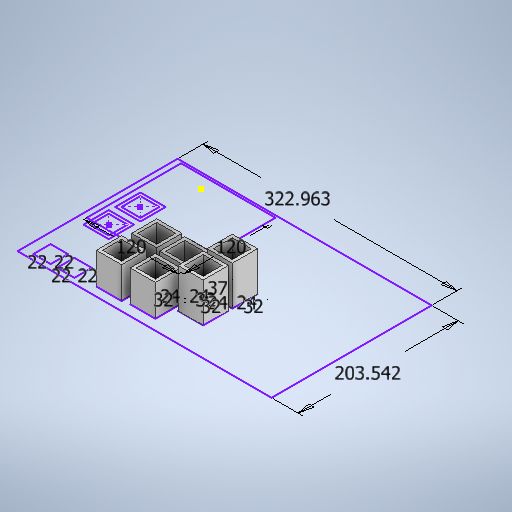
# Autodesk Inventor part: axie3
Saved by Autodesk Inventor 2025.1 (Build 291241000, 241)
## iProperties
Created: 2024-10-25
Part Number: axie3
Material: 一般
Document SubType Name: Modeling
Designer: youtian
Density: 1 g/cm^3
Appearance: 預設
Author: youtian
Autodesk Inventor part; units mm, degrees
ref_plane "YZ Plane" through (0, 0, 0) normal (1, 0, 0) x (0, 1, 0)
ref_plane "XZ Plane" through (0, 0, 0) normal (0, 1, 0) x (-1, 0, 0)
ref_plane "XY Plane" through (0, 0, 0) normal (0, 0, 1) x (1, 0, 0)
sketch "草圖1" plane through (0, 0, 0) normal (0, 1, 0) x (-1, 0, 0)
  circle A0 centre (0, 0) radius 7
  circle A1 centre (0, 0) radius 11
  line L0 (0, 0) -> (-26.517, 0)
  line L1 (0, 0) -> (0, 28.4195)
  circle A2 centre (-26, 0) radius 7
  circle A3 centre (-26, 0) radius 11
  circle A4 centre (0, 26) radius 7
  circle A5 centre (0, 26) radius 11
  circle A6 centre (-26, 26) radius 7
  circle A7 centre (-26, 26) radius 11
  dimension "d0" = 14
  dimension "d1" = 22
  dimension "d6" = 26
  dimension "d9" = 26
  constraints: 8 centre point, 5 coincident, 4 end point, 2 horizontal, 2 vertical, 12 other
  measures "d0" diameter of A0
  measures "d1" diameter of A1
  measures "d6" distance of A0.centre A2.centre
  measures "d9" distance of A0.centre A4.centre
sketch "草圖6" plane through (0, 0, 0) normal (0, 1, 0) x (-1, 0, 0)
  point P0 (0, 0)
sketch "草圖9" plane through (0, 0, 0) normal (0, 1, 0) x (-1, 0, 0)
  line L0 (-119.4877, 79.3379) -> (-151.4877, 79.3379)
  line L1 (-151.4877, 79.3379) -> (-151.4877, 111.3379)
  line L2 (-151.4877, 111.3379) -> (-119.4877, 111.3379)
  line L3 (-119.4877, 111.3379) -> (-119.4877, 79.3379)
  line L4 (-123.4877, 83.3379) -> (-147.4877, 83.3379)
  line L5 (-147.4877, 83.3379) -> (-147.4877, 107.3379)
  line L6 (-147.4877, 107.3379) -> (-123.4877, 107.3379)
  line L7 (-123.4877, 107.3379) -> (-123.4877, 83.3379)
  line L8 (-123.4877, 83.3379) -> (-147.4877, 107.3379) construction
  line L9 (-147.4877, 83.3379) -> (-123.4877, 107.3379) construction
  line L10 (-119.4877, 116.3379) -> (-151.4877, 116.3379)
  line L11 (-151.4877, 116.3379) -> (-151.4877, 148.3379)
  line L12 (-151.4877, 148.3379) -> (-119.4877, 148.3379)
  line L13 (-119.4877, 148.3379) -> (-119.4877, 116.3379)
  line L14 (-123.4877, 120.3379) -> (-147.4877, 120.3379)
  line L15 (-147.4877, 120.3379) -> (-147.4877, 144.3379)
  line L16 (-147.4877, 144.3379) -> (-123.4877, 144.3379)
  line L17 (-123.4877, 144.3379) -> (-123.4877, 120.3379)
  line L18 (-123.4877, 120.3379) -> (-147.4877, 144.3379) construction
  line L19 (-147.4877, 120.3379) -> (-123.4877, 144.3379) construction
  line L20 (-82.0628, 102.3085) -> (-114.0628, 102.3085)
  line L21 (-114.0628, 102.3085) -> (-114.0628, 134.3085)
  line L22 (-114.0628, 134.3085) -> (-82.0628, 134.3085)
  line L23 (-82.0628, 134.3085) -> (-82.0628, 102.3085)
  line L24 (-86.0628, 106.3085) -> (-110.0628, 106.3085)
  line L25 (-110.0628, 106.3085) -> (-110.0628, 130.3085)
  line L26 (-110.0628, 130.3085) -> (-86.0628, 130.3085)
  line L27 (-86.0628, 130.3085) -> (-86.0628, 106.3085)
  line L28 (-86.0628, 102.6348) -> (-110.0628, 126.6348) construction
  line L29 (-110.0628, 102.6348) -> (-86.0628, 126.6348) construction
  line L30 (35.5473, 81.3984) -> (3.5473, 81.3984)
  line L31 (3.5473, 81.3984) -> (3.5473, 113.3984)
  line L32 (3.5473, 113.3984) -> (35.5473, 113.3984)
  line L33 (35.5473, 113.3984) -> (35.5473, 81.3984)
  line L34 (31.5472, 85.3984) -> (7.5472, 85.3984)
  line L35 (7.5472, 85.3984) -> (7.5472, 109.3984)
  line L36 (7.5472, 109.3984) -> (31.5472, 109.3984)
  line L37 (31.5472, 109.3984) -> (31.5472, 85.3984)
  line L38 (31.5472, 85.3984) -> (7.5472, 109.3984) construction
  line L39 (7.5472, 85.3984) -> (31.5472, 109.3984) construction
  line L40 (34.8593, 41.843) -> (2.8593, 41.843)
  line L41 (30.8593, 45.843) -> (6.8593, 45.843)
  line L42 (6.8593, 45.843) -> (6.8593, 69.843)
  line L43 (2.8593, 41.843) -> (2.8593, 73.843)
  line L44 (6.8593, 69.843) -> (30.8593, 69.843)
  line L45 (30.8593, 45.843) -> (6.8593, 69.843) construction
  line L46 (6.8593, 45.843) -> (30.8593, 69.843) construction
  line L47 (2.8593, 73.843) -> (34.8593, 73.843)
  line L48 (30.8593, 69.843) -> (30.8593, 45.843)
  line L49 (34.8593, 73.843) -> (34.8593, 41.843)
  line L50 (-44.571, 100.4659) -> (-76.571, 100.4659)
  line L51 (-48.5711, 104.466) -> (-72.5711, 104.466)
  line L52 (-72.5711, 104.466) -> (-72.5711, 128.466)
  line L53 (-76.571, 100.4659) -> (-76.571, 132.4659)
  line L54 (-72.5711, 128.466) -> (-48.5711, 128.466)
  line L55 (-48.5711, 104.466) -> (-72.5711, 128.466) construction
  line L56 (-72.5711, 104.466) -> (-48.5711, 128.466) construction
  line L57 (-76.571, 132.4659) -> (-44.571, 132.4659)
  line L58 (-48.5711, 128.466) -> (-48.5711, 104.466)
  line L59 (-44.571, 132.4659) -> (-44.571, 100.4659)
  line L60 (-40.805, 141.4327) -> (-72.805, 141.4327)
  line L61 (-44.805, 145.4328) -> (-68.805, 145.4328)
  line L62 (-68.805, 145.4328) -> (-68.805, 169.4328)
  line L63 (-72.805, 141.4327) -> (-72.805, 173.4327)
  line L64 (-68.805, 169.4328) -> (-44.805, 169.4328)
  line L65 (-44.805, 145.4328) -> (-68.805, 169.4328) construction
  line L66 (-68.805, 145.4328) -> (-44.805, 169.4328) construction
  line L67 (-72.805, 173.4327) -> (-40.805, 173.4327)
  line L68 (-44.805, 169.4328) -> (-44.805, 145.4328)
  line L69 (-40.805, 173.4327) -> (-40.805, 141.4327)
  line L70 (-81.8163, 139.4435) -> (-113.8163, 139.4435)
  line L71 (-85.8164, 143.4436) -> (-109.8164, 143.4436)
  line L72 (-109.8164, 143.4436) -> (-109.8164, 167.4436)
  line L73 (-113.8163, 139.4435) -> (-113.8163, 171.4435)
  line L74 (-109.8164, 167.4436) -> (-85.8164, 167.4436)
  line L75 (-85.8164, 143.4436) -> (-109.8164, 167.4436) construction
  line L76 (-109.8164, 143.4436) -> (-85.8164, 167.4436) construction
  line L77 (-113.8163, 171.4435) -> (-81.8163, 171.4435)
  line L78 (-85.8164, 167.4436) -> (-85.8164, 143.4436)
  line L79 (-81.8163, 171.4435) -> (-81.8163, 139.4435)
  point P0 (0, 0)
  point P1 (-135.4877, 95.3379)
  point P2 (-135.4877, 132.3379)
  point P3 (-98.0628, 114.6348)
  point P4 (19.5472, 97.3984)
  point P5 (18.8593, 57.843)
  point P6 (-60.5711, 116.466)
  point P7 (-56.805, 157.4328)
  point P8 (-97.8164, 155.4436)
  dimension "d73" = 50.747
  dimension "d54" = 32
  dimension "d55" = 32
  dimension "d56" = 24
  dimension "d57" = 24
  dimension "d60" = 37
  dimension "d69" = 32
  dimension "d70" = 32
  dimension "d71" = 24
  dimension "d72" = 24
  constraints: 160 end point, 8 parallel, 4 horizontal, 4 midpoint, 4 perpendicular, 2 vertical, 1 collinear, 18 other
  measures "d54" distance of L1.end L2.end
  measures "d55" distance of L0.end L1.end
  measures "d56" distance of L5.end L6.end
  measures "d57" distance of L4.end L5.end
  measures "d60" distance of L0.start L10.start
  measures "d69" distance of L22.start L22.end
  measures "d70" distance of L20.end L22.start
  measures "d71" distance of L26.start L26.end
  measures "d72" distance of L24.end L26.start
extrude "擠出9" add sketch "草圖9" along normal blind 50 contours L0 L1 L2 L3 | L10 L11 L12 L13
extrude "擠出10" add sketch "草圖9" along normal blind 40 contours L20 L21 L22 L23 | L50 L53 L57 L59 | L60 L63 L67 L69 | L70 L73 L77 L79
sketch "草圖10" plane through (0, 0, 0) normal (0, 1, 0) x (-1, 0, 0)
  line L0 (48.2716, 184.5725) -> (-274.6912, 184.5725)
  line L1 (-274.6912, 184.5725) -> (-274.6912, -18.9692)
  line L2 (-274.6912, -18.9692) -> (48.2716, -18.9692)
  line L3 (48.2716, -18.9692) -> (48.2716, 184.5725)
  point P0 (0, 0)
  dimension "d99" = 322.9628
  dimension "d100" = 203.5417
  constraints: 8 end point, 2 parallel, 1 horizontal, 1 perpendicular
  measures "d99" distance of L1.end L2.end
  measures "d100" distance of L0.end L1.end
sketch "草圖11" plane through (0, 0, 0) normal (0, 1, 0) x (-1, 0, 0)
  line L0 (35.0654, 155.7952) -> (13.0654, 155.7952)
  line L1 (13.0654, 155.7952) -> (13.0654, 177.7952)
  line L2 (13.0654, 177.7952) -> (35.0654, 177.7952)
  line L3 (35.0654, 177.7952) -> (35.0654, 155.7952)
  line L4 (4.7905, 155.7952) -> (-17.2095, 155.7952)
  line L5 (-17.2095, 155.7952) -> (-17.2095, 177.7952)
  line L6 (-17.2095, 177.7952) -> (4.7905, 177.7952)
  line L7 (4.7905, 177.7952) -> (4.7905, 155.7952)
  point P0 (0, 0)
  dimension "d101" = 22
  dimension "d102" = 22
  dimension "d103" = 22
  dimension "d104" = 22
  constraints: 16 end point, 4 parallel, 2 horizontal, 2 perpendicular
  measures "d101" distance of L1.end L2.end
  measures "d102" distance of L0.end L1.end
  measures "d103" distance of L5.end L6.end
  measures "d104" distance of L4.end L5.end
sketch "草圖12" plane through (0, 0, 0) normal (0, 1, 0) x (-1, 0, 0)
  line L0 (-109.331, 73.1874) -> (-109.331, 93.1874)
  line L1 (-109.331, 93.1874) -> (-89.331, 93.1874)
  line L2 (-89.331, 93.1874) -> (-89.331, 73.1874)
  line L3 (-89.331, 73.1874) -> (-109.331, 73.1874)
  line L4 (-80.953, 73.904) -> (-80.953, 93.904)
  line L5 (-80.953, 93.904) -> (-60.953, 93.904)
  line L6 (-60.953, 93.904) -> (-60.953, 73.904)
  line L7 (-60.953, 73.904) -> (-80.953, 73.904)
  line L8 (-38.2379, 177.9784) -> (-158.2379, 177.9784)
  line L9 (-158.2379, 177.9784) -> (-158.2379, 57.9784)
  line L10 (-158.2379, 57.9784) -> (-38.2379, 57.9784)
  line L11 (-38.2379, 57.9784) -> (-38.2379, 177.9784)
  point P0 (0, 0)
  dimension "d105" = 20
  dimension "d106" = 20
  dimension "d107" = 20
  dimension "d108" = 20
  dimension "d137" = 120
  dimension "d138" = 120
  constraints: 24 end point, 6 parallel, 3 perpendicular, 1 horizontal
  measures "d105" distance of L1.end L2.end
  measures "d106" distance of L0.end L1.end
  measures "d107" distance of L5.end L6.end
  measures "d108" distance of L4.end L5.end
  measures "d137" distance of L10.end L9.end
  measures "d138" distance of L9.end L8.end
extrude "擠出12" add sketch "草圖12" along normal blind 12 contours L0 L1 L2 L3 | L4 L5 L6 L7
sketch "草圖13" plane through (0, 12, 0) normal (0, 1, 0) x (1, 0, 0)
  line L0 (60.953, -73.904) -> (60.953, -93.904) projected
  line L1 (80.953, -93.904) -> (80.953, -73.904) projected
  line L2 (60.953, -93.904) -> (80.953, -73.904)
  line L3 (89.331, -93.1874) -> (109.331, -93.1874) projected
  line L4 (109.331, -93.1874) -> (109.331, -73.1874) projected
  line L5 (89.331, -93.1874) -> (109.331, -73.1874)
  line L6 (-13.0654, -155.7952) -> (-35.0654, -155.7952) projected
  line L7 (-35.0654, -177.7952) -> (-13.0654, -177.7952) projected
  line L8 (-35.0654, -155.7952) -> (-13.0654, -177.7952)
  line L9 (-4.7905, -177.7952) -> (17.2095, -177.7952) projected
  line L10 (-4.7905, -155.7952) -> (17.2095, -177.7952)
  line L11 (-31.0654, -159.7952) -> (-17.0654, -159.7952)
  line L12 (-17.0654, -159.7952) -> (-17.0654, -173.7952)
  line L13 (-17.0654, -173.7952) -> (-31.0654, -173.7952)
  line L14 (-31.0654, -173.7952) -> (-31.0654, -159.7952)
  line L15 (-31.0654, -159.7952) -> (-17.0654, -173.7952) construction
  line L16 (-17.0654, -159.7952) -> (-31.0654, -173.7952) construction
  line L17 (-0.7905, -173.7952) -> (13.2095, -173.7952)
  line L18 (13.2095, -173.7952) -> (13.2095, -159.7952)
  line L19 (13.2095, -159.7952) -> (-0.7905, -159.7952)
  line L20 (-0.7905, -159.7952) -> (-0.7905, -173.7952)
  line L21 (-0.7905, -173.7952) -> (13.2095, -159.7952) construction
  line L22 (13.2095, -173.7952) -> (-0.7905, -159.7952) construction
  line L23 (65.853, -78.804) -> (76.053, -78.804)
  line L24 (76.053, -78.804) -> (76.053, -89.004)
  line L25 (76.053, -89.004) -> (65.853, -89.004)
  line L26 (65.853, -89.004) -> (65.853, -78.804)
  line L27 (65.853, -78.804) -> (76.053, -89.004) construction
  line L28 (76.053, -78.804) -> (65.853, -89.004) construction
  line L29 (94.231, -88.2874) -> (104.431, -88.2874)
  line L30 (104.431, -88.2874) -> (104.431, -78.0874)
  line L31 (104.431, -78.0874) -> (94.231, -78.0874)
  line L32 (94.231, -78.0874) -> (94.231, -88.2874)
  line L33 (94.231, -88.2874) -> (104.431, -78.0874) construction
  line L34 (104.431, -88.2874) -> (94.231, -78.0874) construction
  point P0 (0, 0)
  point P1 (-24.0654, -166.7952)
  point P2 (6.2095, -166.7952)
  point P3 (70.953, -83.904)
  point P4 (99.331, -83.1874)
  dimension "d113" = 14
  dimension "d114" = 14
  dimension "d115" = 14
  dimension "d116" = 14
  dimension "d117" = 10.2
  dimension "d118" = 10.2
  dimension "d119" = 10.2
  dimension "d120" = 10.2
  constraints: 56 end point, 12 midpoint, 8 parallel, 4 horizontal, 4 perpendicular
  measures "d113" distance of L12.end L13.end
  measures "d114" distance of L11.end L12.end
  measures "d115" distance of L19.end L18.end
  measures "d116" distance of L18.end L17.end
  measures "d117" distance of L24.end L25.end
  measures "d118" distance of L23.end L24.end
  measures "d119" distance of L31.end L30.end
  measures "d120" distance of L30.end L29.end
extrude "擠出13" cut sketch "草圖13" against normal blind 5.6 contours L26 L23 L2 | L2 L24 L25 | L32 L31 L5 | L5 L30 L29 | L11 L12 L8 | L8 L13 L14 | L19 L18 L10 | L10 L17 L20
sketch "草圖15" plane through (0, 0, 0) normal (0, 1, 0) x (-1, 0, 0)
  line L0 (41.1091, -16.1505) -> (-78.8909, -16.1505)
  line L1 (-78.8909, -16.1505) -> (-78.8909, 103.8495)
  line L2 (-78.8909, 103.8495) -> (41.1091, 103.8495)
  line L3 (41.1091, 103.8495) -> (41.1091, -16.1505)
  point P0 (0, 0)
  dimension "d135" = 120
  dimension "d136" = 120
  constraints: 8 end point, 2 parallel, 1 horizontal, 1 perpendicular
  measures "d135" distance of L1.end L2.end
  measures "d136" distance of L0.end L1.end
